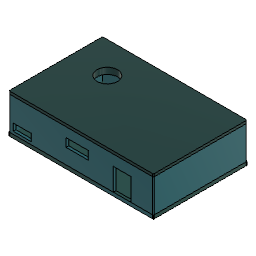
wildfire prediction Device (Autodesk Fusion 360 design; units mm, degrees)
Autodesk Fusion 360 part; units mm, degrees
sketch "Sketch1" plane through (0, 0, 0) normal (0, 0, 1) x (1, 0, 0)
  line L0 (0, 0) -> (162, 0)
  line L1 (162, 0) -> (162, -105)
  line L2 (162, -105) -> (0, -105)
  line L3 (0, -105) -> (0, 0)
  line L4 (3, -8.8701) -> (3, -3)
  line L5 (3, -3) -> (3, -102)
  line L6 (6, -3) -> (3, -3)
  line L7 (3, -3) -> (159, -3)
  line L8 (159, -6) -> (159, -3)
  line L9 (159, -3) -> (159, -102)
  line L10 (158, -102) -> (162, -102)
  line L11 (159, -102) -> (3, -102)
  line L12 (29.6, -18.6883) -> (29.6, -3)
  line L13 (29.6, -3) -> (29.6, -63)
  line L14 (84.5, -11.142) -> (84.5, -3)
  line L15 (84.5, -3) -> (84.5, -63)
  line L16 (29.6, -63) -> (84.5, -63)
  line L17 (143, -6) -> (143, -3)
  line L18 (143, -3) -> (143, -26.5)
  line L19 (132.5048, -26.5) -> (143, -26.5)
  line L20 (123, -11) -> (123, -3)
  line L21 (123, -11) -> (123, -26.5)
  line L22 (132.5048, -26.5) -> (123, -26.5)
  dimension "d1" = 162
  dimension "d2" = 105
  dimension "d23" = 60
  dimension "d25" = 16
  constraint coincident L0.start L3.end
  constraint horizontal L0
  constraint perpendicular L0 L1
  constraint perpendicular L1 L2
  constraint perpendicular L0 L3
  constraint perpendicular L0 L4
  constraint perpendicular L2 L5
  constraint perpendicular L3 L6
  constraint perpendicular L1 L7
  constraint perpendicular L0 L8
  constraint perpendicular L2 L9
  constraint coincident L1 L10.end
  constraint perpendicular L1 L10
  constraint perpendicular L3 L11
  constraint coincident L7 L12.end
  constraint perpendicular L7 L12
  constraint perpendicular L7 L13
  constraint coincident L7 L14.end
  constraint perpendicular L7 L14
  constraint perpendicular L7 L15
  constraint coincident L15 L16.end
  constraint perpendicular L15 L16
  constraint coincident L7 L17.end
  constraint perpendicular L7 L17
  constraint perpendicular L7 L18
  constraint perpendicular L18 L19
  constraint coincident L7 L20.end
  constraint perpendicular L7 L20
  constraint perpendicular L21 L22
  measures "d1" distance of L0.start L0.end
  measures "d2" distance of L0.end L1.end
  measures "d23" distance of L12.end L13.end
  measures "d25" distance of L8.start L17.start
extrude "Extrude1" add sketch "Sketch1" along normal blind 4 contours L0 L1 L2 L3 | L4 L5 L6 L7 L8 L9 L10 L11 L12 L13 L14 L15 L16 L17 L18 L19 L20 L21 L22 makes body 1
extrude "Extrude3" add sketch "Sketch1" along normal blind 41 separate body makes body 2
sketch "Sketch3" plane through (0, 0, 0) normal (0, 0, 1) x (1, 0, 0)
  line L0 (3.3483, 144.9883) -> (165.3483, 144.9883)
  line L1 (165.3483, 144.9883) -> (165.3483, 39.9883)
  line L2 (165.3483, 39.9883) -> (3.3483, 39.9883)
  line L3 (3.3483, 39.9883) -> (3.3483, 144.9883)
  line L4 (6.3288, 142.5582) -> (161.8288, 142.5582)
  line L5 (161.8288, 142.5582) -> (161.8288, 44.0582)
  line L6 (161.8288, 44.0582) -> (6.3288, 44.0582)
  line L7 (6.3288, 44.0582) -> (6.3288, 142.5582)
  dimension "d29" = 162
  dimension "d30" = 105
  dimension "d31" = 155.5
  dimension "d32" = 98.5
  constraint horizontal L0
  constraint vertical L1
  constraint horizontal L2
  constraint vertical L3
  constraint horizontal L4
  constraint vertical L5
  constraint horizontal L6
  constraint vertical L7
  measures "d29" distance of L0.start L0.end
  measures "d30" distance of L0.start L2.end
  measures "d31" distance of L4.start L4.end
  measures "d32" distance of L4.start L6.end
extrude "Extrude4" add sketch "Sketch3" along normal blind 7 separate body contours L4 L5 L6 L7 makes body 3
extrude "Extrude5" add sketch "Sketch3" along normal blind 3 bodies 3
sketch "Sketch4" plane through (0, 0, 0) normal (0, 1, 0) x (-1, 0, 0)
  line L0 (-162, 0) -> (0, 0)
  line L1 (0, 0) -> (0, 41)
  line L2 (0, 41) -> (-162, 41)
  line L3 (-162, 41) -> (-162, 0)
move_body "Move1" bodies 3 to x (1, 0, 0) y (0, 1, 0) z (0, 0, 1) at (-5, 0, 0)
sketch "Sketch5" plane through (0, 0, 0) normal (0, 1, 0) x (-1, 0, 0)
sketch "Sketch6" plane through (0, 0, 0) normal (0, 1, 0) x (-1, 0, 0)
  line L0 (-60, 16) -> (-60, 3)
  line L1 (-115, 16) -> (-95, 16)
  line L2 (-95, 16) -> (-95, 11)
  line L3 (-95, 11) -> (-115, 11)
  line L4 (-115, 11) -> (-115, 16)
  line L5 (-60, 16) -> (-80, 16)
  line L6 (-80, 16) -> (-80, 3)
  line L7 (-80, 3) -> (-60, 3)
  line L8 (-60, 3) -> (-60, 16)
  line L9 (-95, 3) -> (-115, 3)
  line L10 (-115, 3) -> (-115, 6)
  line L11 (-115, 6) -> (-95, 6)
  line L12 (-95, 6) -> (-95, 3)
  line L13 (-115, 16) -> (-95, 16)
  line L14 (-80, 16) -> (-60, 16)
  line L15 (-115, 16) -> (-115, 11)
  line L16 (-115, 6) -> (-115, 3)
  dimension "d38" = 55
  constraint perpendicular L0 L13
  constraint horizontal L1
  constraint vertical L2
  constraint horizontal L3
  constraint vertical L4
  constraint horizontal L5
  constraint vertical L6
  constraint horizontal L7
  constraint vertical L8
  constraint horizontal L9
  constraint vertical L10
  constraint horizontal L11
  constraint vertical L12
  constraint coincident L10.end L15
  constraint collinear L13 L14
  constraint collinear L15 L16
  measures "d38" distance of L1.start L0.start
extrude "Extrude6" cut sketch "Sketch6" against normal blind 5 bodies 1 2
sketch "Sketch7" plane through (0, -105, 0) normal (0, -1, 0) x (1, 0, 0)
  line L0 (0, 0) -> (162, 0)
  line L1 (162, 0) -> (162, 41)
  line L2 (162, 41) -> (0, 41)
  line L3 (0, 41) -> (0, 0)
  line L4 (117, 4) -> (117, 29)
  line L5 (117, 29) -> (137, 29)
  line L6 (137, 29) -> (137, 4)
  line L7 (137, 4) -> (117, 4)
  line L8 (89, 21) -> (64.1, 21)
  line L9 (64.1, 30.4402) -> (89, 30.4402)
  line L10 (89, 30.4402) -> (89, 21)
  line L11 (88, 30.4402) -> (64.1, 30.4402)
  line L12 (64.1, 30.4402) -> (64.1, 21)
  line L13 (5, 15) -> (25, 15)
  line L14 (25, 15) -> (25, 7)
  line L15 (25, 7) -> (5, 7)
  line L16 (5, 7) -> (5, 15)
  dimension "d46" = 24.9
  constraint vertical L4
  constraint perpendicular L5 L6
  constraint perpendicular L4 L7
  constraint coincident L9 L11.start
  constraint perpendicular L8 L12
  constraint horizontal L13
  constraint vertical L14
  constraint horizontal L15
  constraint vertical L16
  measures "d46" distance of L8.start L8.end
extrude "Extrude7" cut sketch "Sketch7" against normal blind 5 contours L4 L5 L6 L7 | L8 L9 L10 L11 L12 | L13 L14 L15 L16 bodies 2
sketch "Top Part" plane through (0, 0, 7) normal (0, 0, 1) x (-1, 0, 0)
  line L0 (-1.3288, -44.0582) -> (-156.8288, -44.0582)
  line L1 (-156.8288, -44.0582) -> (-156.8288, -142.5582)
  line L2 (-156.8288, -142.5582) -> (-1.3288, -142.5582)
  line L3 (-1.3288, -142.5582) -> (-1.3288, -44.0582)
  line L4 (-33.744, -64.9559) -> (-33.8288, -64.9559)
  circle A0 centre (-38.899, -75.2038) radius 11.4714
  circle A1 centre (-22.3288, -130.5582) radius 10
  line L5 (-6.3288, -142.5582) -> (-161.8288, -142.5582)
  line L6 (-6.3288, -44.0582) -> (-6.3288, -142.5582)
  line L7 (-70.745, -135.77) -> (-85.745, -135.77)
  line L8 (-85.745, -135.77) -> (-85.745, -110.77)
  line L9 (-85.745, -110.77) -> (-70.745, -110.77)
  line L10 (-70.745, -110.77) -> (-70.745, -135.77)
  line L11 (-85.745, -123.27) -> (-70.745, -123.27)
  circle A2 centre (-78.245, -123.27) radius 7.4728
  line L12 (-94.4278, -134.7092) -> (-124.4278, -134.7092)
  line L13 (-124.4278, -134.7092) -> (-124.4278, -94.7092)
  line L14 (-124.4278, -94.7092) -> (-94.4278, -94.7092)
  line L15 (-94.4278, -94.7092) -> (-94.4278, -134.7092)
  circle A3 centre (-109.4278, -114.7092) radius 15
  line L16 (-91.8288, -79.0582) -> (-106.8288, -79.0582)
  line L17 (-106.8288, -79.0582) -> (-106.8288, -54.0582)
  line L18 (-106.8288, -54.0582) -> (-91.8288, -54.0582)
  line L19 (-91.8288, -54.0582) -> (-91.8288, -79.0582)
  circle A4 centre (-99.3288, -66.5582) radius 7.5
  line L20 (-161.8288, -44.0582) -> (-6.3288, -44.0582)
  dimension "d78" = 20
  dimension "d79" = 12
  dimension "d80" = 16
  dimension "d81" = 15
  dimension "d82" = 25
  dimension "d83" = 30
  dimension "d84" = 40
  dimension "d85" = 30
  dimension "d86" = 15
  dimension "d87" = 20
  dimension "d88" = 15
  dimension "d89" = 25
  dimension "d90" = 15
  dimension "d91" = 7.5
  dimension "d92" = 12.5
  dimension "d93" = 50
  dimension "d94" = 10
  constraint perpendicular L3 L4
  constraint coincident A0 L4.start
  constraint horizontal L7
  constraint vertical L8
  constraint horizontal L9
  constraint vertical L10
  constraint midpoint L8 L11.start
  constraint midpoint L10 L11.end
  constraint horizontal L12
  constraint vertical L13
  constraint horizontal L14
  constraint vertical L15
  constraint horizontal L16
  constraint vertical L17
  constraint horizontal L18
  constraint vertical L19
  measures "d78" diameter of A1
  measures "d79" distance of A1.centre L5
  measures "d80" distance of A1.centre L6
  measures "d81" distance of L7.start L7.end
  measures "d82" distance of L7.start L9.end
  measures "d83" distance of L12.start L12.end
  measures "d84" distance of L12.start L14.end
  measures "d85" diameter of A3
  measures "d86" distance of L15 A3.centre
  measures "d87" distance of L12 A3.centre
  measures "d88" distance of L16.start L16.end
  measures "d89" distance of L16.start L18.end
  measures "d90" diameter of A4
  measures "d91" distance of L19 A4.centre
  measures "d92" distance of L16 A4.centre
  measures "d93" distance of L1 L17
  measures "d94" distance of L18 L20
extrude "Extrude9" cut sketch "Top Part" against normal blind 30 contours A0 bodies 3
fillet "Fillet1" radius 1 1 edges at (29.6, -33, 0) on bodies 1
fillet "Fillet2" radius 1 2 edges at (29.3071, -63, 0.2929) (29.6, -63, 2.5) on bodies 1
fillet "Fillet3" radius 1 1 edges at (84.5, -63, 2) on bodies 1
fillet "Fillet4" radius 1 1 edges at (84.5, -3, 2) on bodies 1
fillet "Fillet5" radius 1 2 edges at (29.3071, -3, 0.2929) (29.6, -3, 2.5) on bodies 1
fillet "Fillet6" radius 1 1 edges at (0, 0, 20.5) on bodies 2
fillet "Fillet7" radius 1 2 edges at (0, -105, 20.5) (162, -105, 20.5) on bodies 2
fillet "Fillet8" radius 1 1 edges at (162, 0, 20.5) on bodies 2
fillet "Fillet9" radius 1 4 edges at (160.3483, 39.9883, 1.5) (160.3483, 144.9883, 1.5) (-1.6517, 144.9883, 1.5) (-1.6517, 39.9883, 1.5) on bodies 3
copy_body "Body->Comp1" bodies 3 removing the originals makes body 4 in component "Component"
extrude "Extrude8" [suppressed]
component "Component" placed x (1, 0, 0) y (0, -1, 0) z (0, 0, -1) at (1.6517, 39.9883, 44)
equation "d79 = 2 mm + ( d78 / 2 )"
equation "d80 = 6 mm + ( d78 / 2 )"
equation "d85 = d83"
equation "d86 = d83 / 2"
equation "d87 = d84 / 2"
equation "d90 = d88"
equation "d91 = d88 / 2"
equation "d92 = d89 / 2"
